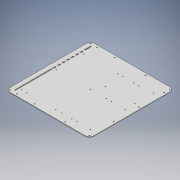
# Autodesk Inventor part: right_panel2
Saved by Autodesk Inventor 2018 (Build 220112000, 112)
## iProperties
Created: 2021-05-09
Part Number: right_panel2
Material: Generic
Document SubType Name: Modeling
Designer: gisen
Density: 1 g/cm^3
Appearance: Default
Author: gisen
Autodesk Inventor part; units mm, degrees
ref_plane "YZ Plane" through (0, 0, 0) normal (1, 0, 0) x (0, 1, 0)
ref_plane "XZ Plane" through (0, 0, 0) normal (0, 1, 0) x (-1, 0, 0)
ref_plane "XY Plane" through (0, 0, 0) normal (0, 0, 1) x (1, 0, 0)
sketch "Sketch1" plane through (0, 0, 0) normal (0, 0, 1) x (1, 0, 0)
  circle A0 centre (95.9523, -199.0135) radius 1.6
  circle A1 centre (-154.2377, -199.0135) radius 1.6
  circle A2 centre (23.5623, 4.1865) radius 1.6
  circle A3 centre (158.1823, -41.5335) radius 1.6
  circle A4 centre (95.9523, 82.9265) radius 1.6
  circle A5 centre (158.1823, 88.0065) radius 1.6
  circle A6 centre (158.1823, 4.1865) radius 1.6
  circle A7 centre (158.1823, -198.9135) radius 1.6
  circle A8 centre (23.5623, 82.9265) radius 1.6
  circle A9 centre (95.9523, -41.5335) radius 1.6
  circle A10 centre (27.3723, -199.0135) radius 1.6
  circle A11 centre (70, 139.5002) radius 2.25
  circle A12 centre (180, -115) radius 2.25
  circle A13 centre (-70, 139.5002) radius 2.25
  circle A14 centre (70, -225) radius 2.25
  circle A15 centre (-70, -225) radius 2.25
  circle A16 centre (180, 0) radius 2.25
  circle A17 centre (180, 115) radius 2.25
  line L0 (-170.25, 129.7502) -> (-166.75, 129.7502)
  line L1 (-170.25, -10.0108) -> (-165.75, -10.0108)
  line L2 (-165.75, -10.0108) -> (-165.75, -20.7978)
  line L3 (-165.75, -20.7978) -> (-170.25, -20.7978)
  line L4 (-170.25, -20.7978) -> (-170.25, -10.0108)
  line L5 (-170.25, 30.9892) -> (-165.75, 30.9892)
  line L6 (-165.75, 30.9892) -> (-165.75, 20.2022)
  line L7 (-165.75, 20.2022) -> (-170.25, 20.2022)
  line L8 (-170.25, 20.2022) -> (-170.25, 30.9892)
  line L9 (-170.25, 71.9892) -> (-165.75, 71.9892)
  line L10 (-165.75, 71.9892) -> (-165.75, 61.2022)
  line L11 (-165.75, 61.2022) -> (-170.25, 61.2022)
  line L12 (-170.25, 61.2022) -> (-170.25, 71.9892)
  line L13 (-165.75, 112.9892) -> (-165.75, 102.2022)
  line L14 (-165.75, 102.2022) -> (-170.25, 102.2022)
  line L15 (-170.25, 102.2022) -> (-170.25, 112.9892)
  line L16 (-170.25, 92.6438) -> (-165.75, 92.6438)
  line L17 (-165.75, 92.6438) -> (-165.75, 81.8568)
  line L18 (-165.75, 81.8568) -> (-170.25, 81.8568)
  line L19 (-170.25, 81.8568) -> (-170.25, 92.6438)
  line L20 (-170.25, 51.6438) -> (-165.75, 51.6438)
  line L21 (-165.75, 51.6438) -> (-165.75, 40.8568)
  line L22 (-165.75, 40.8568) -> (-170.25, 40.8568)
  line L23 (-170.25, 40.8568) -> (-170.25, 51.6438)
  line L24 (-170.25, 10.6438) -> (-165.75, 10.6438)
  line L25 (-165.75, 10.6438) -> (-165.75, -0.1432)
  line L26 (-165.75, -0.1432) -> (-170.25, -0.1432)
  line L27 (-170.25, -0.1432) -> (-170.25, 10.6438)
  line L28 (-170.25, -30.3562) -> (-165.75, -30.3562)
  line L29 (-165.75, -30.3562) -> (-165.75, -41.1432)
  line L30 (-165.75, -41.1432) -> (-170.25, -41.1432)
  line L31 (-170.25, -41.1432) -> (-170.25, -30.3562)
  line L32 (-170.25, -215.25) -> (-170.25, -45.8135)
  line L33 (-170.25, -45.8135) -> (-166.75, -45.8135)
  line L34 (-166.75, -45.8135) -> (-166.75, -215.25)
  line L35 (-166.75, -215.25) -> (-170.25, -215.25)
  circle A18 centre (-150, -225) radius 2.25
  circle A19 centre (-150, 139.5002) radius 2.25
  circle A20 centre (73.0923, -41.5335) radius 1.6
  circle A21 centre (0.7023, -199.0135) radius 1.6
  circle A22 centre (-154.2377, -41.5335) radius 1.6
  circle A23 centre (0.7023, 82.9265) radius 1.6
  circle A24 centre (73.0923, 82.9265) radius 1.6
  circle A25 centre (-154.2377, 82.9265) radius 1.6
  circle A26 centre (-131.3777, -199.0135) radius 1.6
  circle A27 centre (73.0923, -199.0135) radius 1.6
  circle A28 centre (0.7023, -41.5335) radius 1.6
  circle A29 centre (180, -225) radius 2.25
  circle A30 centre (-180, -225) radius 2.25
  circle A31 centre (180, 139.5002) radius 2.25
  circle A32 centre (-180, 139.5002) radius 2.25
  line L36 (170, 149.5002) -> (-170, 149.5002)
  arc A33 (-170, 149.5002) -> (-190, 129.5002) centre (-170, 129.5002) ccw
  line L37 (-190, 124.35) -> (-190, -215)
  arc A34 (-190, -215) -> (-170, -235) centre (-170, -215) ccw
  line L38 (-170, -235) -> (170, -235)
  arc A35 (170, -235) -> (190, -215) centre (170, -215) ccw
  line L39 (190, -215) -> (190, 124.35)
  arc A36 (190, 129.5002) -> (170, 149.5002) centre (170, 129.5002) ccw
  line L40 (-190, 129.5002) -> (-190, 124.35)
  line L41 (190, 129.5002) -> (190, 124.35)
  line L42 (-165.75, 112.9892) -> (-165.75, 129.7502)
  line L43 (-165.75, 129.7502) -> (-166.75, 129.7502)
  line L44 (-170.25, 129.7502) -> (-170.25, 112.9892)
  point P0 (0, 0)
  point P1 (0, 0)
  dimension "d197" = 27.548
  constraints: 90 end point, 37 centre point, 8 point on circle, 3 vertical, 1 parallel, 1 perpendicular
  measures "d197" distance between parallel lines of L14 L0
extrude "Extrusion1" add sketch "Sketch1" along normal blind 3
body "Solid1"
